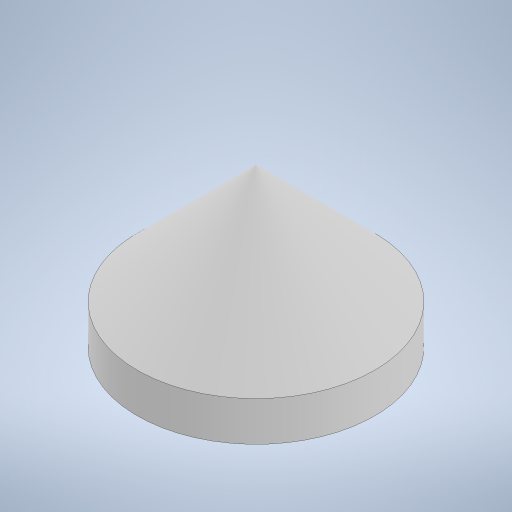
# Autodesk Inventor part: Goma tacómetro_v2
Saved by Autodesk Inventor 2023 (Build 270158000, 158)
## iProperties
Created: 2023-07-25
Part Number: Goma tacómetro_v2
Material: Generic
Document SubType Name: Modeling
Designer: checo
Density: 1 g/cm^3
Appearance: Default
Author: checo
Autodesk Inventor part; units mm, degrees
ref_plane "YZ Plane" through (0, 0, 0) normal (1, 0, 0) x (0, 1, 0)
ref_plane "XZ Plane" through (0, 0, 0) normal (0, 1, 0) x (-1, 0, 0)
ref_plane "XY Plane" through (0, 0, 0) normal (0, 0, 1) x (1, 0, 0)
sketch "Sketch1" plane through (0, 0, 0) normal (0, 1, 0) x (-1, 0, 0)
  circle A0 centre (0, 0) radius 7.5
  circle A1 centre (0, 0) radius 4.75
  circle A2 centre (0, 0) radius 14.25
  circle A3 centre (0, 0) radius 16.5
  line L0 (-4.6435, -1) -> (-7.433, -1)
  line L1 (0, 0) -> (-16.5, 0) construction
  line L2 (-4.6435, 1) -> (-7.433, 1)
  line L3 (1, -4.6435) -> (1, -7.433)
  line L4 (-1, -4.6435) -> (-1, -7.433)
  line L5 (4.6435, 1) -> (7.433, 1)
  line L6 (4.6435, -1) -> (7.433, -1)
  line L7 (-1, 4.6435) -> (-1, 7.433)
  line L8 (1, 4.6435) -> (1, 7.433)
  dimension "d1" = 15
  dimension "d2" = 9.5
  dimension "d3" = 33
  dimension "d0" = 28.5
  dimension "d7" = 1
  dimension "d10" = 360
  constraints: 18 end point, 4 coincident, 2 horizontal, 2 symmetric about line, 1 centre point, 1 horizontal alignment, 33 other
  measures "d0" diameter of A2
  measures "d7" distance from line of point (0, 0) L0
extrude "Extrusion1" add sketch "Sketch1" against normal blind 6 contours A3
extrude "Extrusion2" add sketch "Sketch1" along normal blind 6 contours L5 A1 L8 A0 | A0 L3 A1 L6 | L7 A1 L2 A0 | A0 L0 A1 L4 | A2 | A3
sketch "Sketch2" plane through (0, 6, 0) normal (0, 1, 0) x (1, 0, 0)
  circle A0 centre (0, 0) radius 16.5 projected
extrude "Extrusion3" add sketch "Sketch2" along normal blind 10
chamfer "Chamfer1" distance 16.5 angle 45 1 edges at (-16.5, 16, 0)
body "Solid1"
